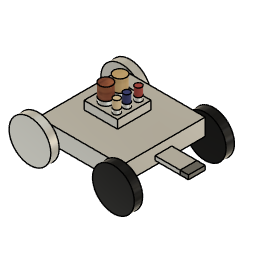
s1100853final (Autodesk Fusion 360 design; units mm, degrees)
Autodesk Fusion 360 part; units mm, degrees
note: some values were not read from the file. Set by a fixed rule: which sketch regions a step uses.
sketch "Sketch1" plane through (0, 0, 0) normal (0, 0, 1) x (1, 0, 0)
  line L0 (0, 0) -> (-100, 0)
  line L1 (-100, 0) -> (-100, -100)
  line L2 (-100, -100) -> (0, -100)
  line L3 (0, -100) -> (0, 0)
  dimension "d1" = 100
  dimension "d2" = 100
  constraint horizontal L0
  constraint vertical L1
  constraint horizontal L2
  constraint vertical L3
  constraint coincident L0.start L3.end
  measures "d1" distance of L0.start L0.end
  measures "d2" distance of L0.start L2.end
extrude "Extrude1" add sketch "Sketch1" along normal blind 20 makes body 1
sketch "Sketch2" plane through (0, 0, 0) normal (0, 1, 0) x (-1, 0, 0)
  line L0 (0, 0) -> (100, 0)
  line L1 (100, 0) -> (100, 20)
  line L2 (100, 20) -> (0, 20)
  line L3 (0, 20) -> (0, 0)
  circle A0 centre (0, 0) radius 25
  dimension "d5" = 50
  constraint coincident L0.start L3.end
  measures "d5" diameter of A0
extrude "Extrude2" add sketch "Sketch2" along normal blind 10 separate body contours L0 L2 L3 A0 | L0 L2 L3 A0 makes body 2
sketch "Sketch3" plane through (0, 0, 0) normal (0, 1, 0) x (-1, 0, 0)
  line L0 (0, 0) -> (100, 0)
  line L1 (100, 0) -> (100, 20)
  line L2 (100, 20) -> (0, 20)
  line L3 (0, 20) -> (0, 0)
  circle A0 centre (100, 0) radius 25
  dimension "d8" = 50
  constraint coincident L0.end L1.start
  measures "d8" diameter of A0
extrude "Extrude3" add sketch "Sketch3" along normal blind 10 contours L0 L1 L2 A0 | L0 L1 L2 A0 bodies 1
sketch "Sketch4" plane through (0, -100, 0) normal (0, -1, 0) x (1, 0, 0)
  line L0 (-100, 0) -> (0, 0)
  line L1 (0, 0) -> (0, 20)
  line L2 (0, 20) -> (-100, 20)
  line L3 (-100, 20) -> (-100, 0)
  circle A0 centre (-100, 0) radius 25
  dimension "d11" = 50
  constraint coincident L0.start L3.end
  measures "d11" diameter of A0
extrude "Extrude4" add sketch "Sketch4" along normal blind 10 contours L0 L2 L3 A0 | L0 L2 L3 A0 bodies 1
sketch "Sketch5" plane through (0, -100, 0) normal (0, -1, 0) x (1, 0, 0)
  arc A0 (-75, 0) -> (-85, 20) centre (-100, 0) ccw
  line L0 (-75, 0) -> (0, 0)
  line L1 (0, 0) -> (0, 20)
  line L2 (0, 20) -> (-85, 20)
  circle A1 centre (0, 0) radius 25
  dimension "d14" = 50
  constraint coincident L0.end L1.start
  measures "d14" diameter of A1
extrude "Extrude5" add sketch "Sketch5" along normal blind 10 separate body contours L0 L1 L2 A1 | L0 L1 L2 A1 makes body 3
move_body "Move1" bodies 2 1 3 to x (1, 0, 0) y (0, 1, 0) z (0, 0, 1) at (0, 0, 25)
sketch "Sketch6" plane through (0, 0, 0) normal (1, 0, 0) x (0, 1, 0)
  line L0 (-100, 25) -> (0, 25)
  line L1 (0, 25) -> (0, 45)
  line L2 (0, 45) -> (-100, 45)
  line L3 (-100, 45) -> (-100, 25)
  line L4 (-60, 35) -> (-40, 35)
  line L5 (-40, 35) -> (-40, 30)
  line L6 (-40, 30) -> (-60, 30)
  line L7 (-60, 30) -> (-60, 35)
  constraint horizontal L4
  constraint vertical L5
  constraint horizontal L6
  constraint vertical L7
extrude "Extrude6" add sketch "Sketch6" along normal blind 30 contours L4 L5 L6 L7 bodies 1
extrude "Extrude7" add 1 faces at (30, -53.3333, 33.3333) along direction (1, 0, 0) blind 10 separate body on bodies 1 makes body 4
sketch "Sketch7" plane through (0, 0, 45) normal (0, 0, 1) x (-1, 0, 0)
  line L0 (0, 100) -> (0, 0)
  line L1 (0, 0) -> (85, 0)
  line L2 (85, 0) -> (100, 0)
  line L3 (100, 0) -> (100, 100)
  line L4 (100, 100) -> (85, 100)
  line L5 (85, 100) -> (0, 100)
  line L6 (40, 65) -> (80, 65)
  line L7 (80, 65) -> (80, 25)
  line L8 (80, 25) -> (40, 25)
  line L9 (40, 25) -> (40, 65)
  dimension "d21" = 40
  dimension "d22" = 40
  constraint horizontal L6
  constraint vertical L7
  constraint horizontal L8
  constraint vertical L9
  measures "d21" distance of L6.start L6.end
  measures "d22" distance of L6.start L8.end
extrude "Extrude8" add sketch "Sketch7" along normal blind 10 contours L6 L7 L8 L9 bodies 1
sketch "Sketch8" plane through (0, 0, 55) normal (0, 0, 1) x (-1, 0, 0)
  line L0 (40, 25) -> (80, 25)
  line L1 (80, 25) -> (80, 65)
  line L2 (80, 65) -> (40, 65)
  line L3 (40, 65) -> (40, 25)
  circle A0 centre (48, 58) radius 4
  dimension "d25" = 8
  measures "d25" diameter of A0
extrude "Extrude9" add sketch "Sketch8" along normal blind 5 contours A0 bodies 1
extrude "Extrude10" add 1 faces at (-46.7702, -57.8013, 60) along direction (0, 0, 1) blind 10 separate body on bodies 1 makes body 5
sketch "Sketch9" plane through (0, 0, 55) normal (0, 0, 1) x (-1, 0, 0)
  circle A0 centre (48, 58) radius 4
  line L0 (40, 25) -> (80, 25)
  line L1 (80, 25) -> (80, 65)
  line L2 (80, 65) -> (40, 65)
  line L3 (40, 65) -> (40, 25)
  circle A1 centre (48, 46) radius 4
  dimension "d30" = 8
  measures "d30" diameter of A1
extrude "Extrude11" add sketch "Sketch9" along normal blind 5 contours A1 bodies 1
extrude "Extrude12" add 1 faces at (-46.7702, -45.8013, 60) along direction (0, 0, 1) blind 10 separate body on bodies 1 makes body 6
sketch "Sketch10" plane through (0, 0, 55) normal (0, 0, 1) x (-1, 0, 0)
  circle A0 centre (48, 46) radius 4
  circle A1 centre (48, 58) radius 4
  line L0 (40, 25) -> (80, 25)
  line L1 (80, 25) -> (80, 65)
  line L2 (80, 65) -> (40, 65)
  line L3 (40, 65) -> (40, 25)
  circle A2 centre (48, 32) radius 4
  dimension "d35" = 8
  measures "d35" diameter of A2
extrude "Extrude13" add sketch "Sketch10" along normal blind 5 contours A2 bodies 1
extrude "Extrude14" add 1 faces at (-46.7702, -31.8013, 60) along direction (0, 0, 1) blind 10 separate body on bodies 1 makes body 7
sketch "Sketch11" plane through (0, 0, 55) normal (0, 0, 1) x (-1, 0, 0)
  circle A0 centre (48, 32) radius 4
  circle A1 centre (48, 46) radius 4
  circle A2 centre (48, 58) radius 4
  line L0 (40, 25) -> (80, 25)
  line L1 (80, 25) -> (80, 65)
  line L2 (80, 65) -> (40, 65)
  line L3 (40, 65) -> (40, 25)
  circle A3 centre (66, 53) radius 7.5
  dimension "d40" = 15
  measures "d40" diameter of A3
extrude "Extrude15" add sketch "Sketch11" along normal blind 5 contours A3 bodies 1
extrude "Extrude16" add 1 faces at (-70.5871, -52.8899, 60) along direction (0, 0, 1) blind 15 separate body on bodies 1 makes body 8
sketch "Sketch12" plane through (0, 0, 55) normal (0, 0, 1) x (-1, 0, 0)
  circle A0 centre (66, 53) radius 7.5
  circle A1 centre (48, 32) radius 4
  circle A2 centre (48, 46) radius 4
  circle A3 centre (48, 58) radius 4
  line L0 (40, 25) -> (80, 25)
  line L1 (80, 25) -> (80, 65)
  line L2 (80, 65) -> (40, 65)
  line L3 (40, 65) -> (40, 25)
  circle A4 centre (66, 36) radius 7.5
  dimension "d45" = 15
  measures "d45" diameter of A4
extrude "Extrude17" add sketch "Sketch12" along normal blind 5 contours A4 bodies 1
extrude "Extrude18" add 1 faces at (-62.2779, -37.1948, 60) along direction (0, 0, 1) blind 15 separate body on bodies 1 makes body 9
copy_body "Body->Comp1" bodies 1 removing the originals makes body 10 in component "base_link"
copy_body "Body->Comp2" bodies 2 removing the originals makes body 11 in component "left_wheel"
copy_body "Body->Comp3" bodies 3 removing the originals makes body 12 in component "right_wheel"
copy_body "Body->Comp4" bodies 4 removing the originals makes body 13 in component "Bumper"
copy_body "Body->Comp5" bodies 5 removing the originals makes body 14 in component "Lidar"
copy_body "Body->Comp6" bodies 6 removing the originals makes body 15 in component "Depth_Camera"
copy_body "Body->Comp7" bodies 7 removing the originals makes body 16 in component "Camera"
copy_body "Body->Comp8" bodies 8 removing the originals makes body 17 in component "IMU"
copy_body "Body->Comp9" bodies 9 removing the originals makes body 18 in component "GPS"
component "base_link" placed x (1, 0, 0) y (0, 1, 0) z (0, 0, 1) at (0, 0, 0)
component "left_wheel" placed x (1, 0, 0) y (0, 1, 0) z (0, 0, 1) at (0, 0, 0)
component "right_wheel" placed x (1, 0, 0) y (0, 1, 0) z (0, 0, 1) at (0, 0, 0)
component "Bumper" placed x (1, 0, 0) y (0, 1, 0) z (0, 0, 1) at (0, 0, 0)
component "Lidar" placed x (1, 0, 0) y (0, 1, 0) z (0, 0, 1) at (0, 0, 0)
component "Depth_Camera" placed x (1, 0, 0) y (0, 1, 0) z (0, 0, 1) at (0, 0, 0)
component "Camera" placed x (1, 0, 0) y (0, 1, 0) z (0, 0, 1) at (0, 0, 0)
component "IMU" placed x (1, 0, 0) y (0, 1, 0) z (0, 0, 1) at (0, 0, 0)
component "GPS" placed x (1, 0, 0) y (0, 1, 0) z (0, 0, 1) at (0, 0, 0)
named bodies: "base_link", "right_wheel", "left_wheel", "Bumper", "Lidar", "Depth_Camera", "Camera", "IMU", "GPS"
